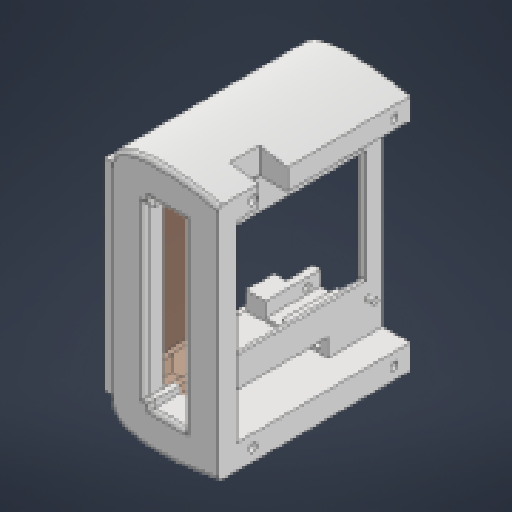
# Autodesk Inventor part: BP_BackHSCover
Saved by Autodesk Inventor 2026.1 (Build 301233020, 233B)
## iProperties
Created: 2025-09-12
Part Number: BP_BackHSCover
Material: Generic
Document SubType Name: Modeling
Designer: atrus
Density: 1 g/cm^3
Appearance: Default
Author: atrus
Autodesk Inventor part; units mm, degrees
ref_plane "YZ Plane" through (0, 0, 0) normal (1, 0, 0) x (0, 1, 0)
ref_plane "XZ Plane" through (0, 0, 0) normal (0, 1, 0) x (-1, 0, 0)
ref_plane "XY Plane" through (0, 0, 0) normal (0, 0, 1) x (1, 0, 0)
ref_plane "Work Plane1" through (0, 0, 0) normal (0, 0, 1) x (1, 0, 0)
sketch "Sketch1" plane through (0, 0, 0) normal (0, 0, 1) x (1, 0, 0)
  line L0 (-13.535, 44.65) -> (-5.515, 44.65)
  line L1 (-13.535, 37.45) -> (-13.535, 44.65)
  line L2 (-5.515, 44.65) -> (-5.515, 41.182512)
  line L3 (-5.515, 41.182512) -> (-2.515, 41.182512)
  line L4 (-2.515, 41.182512) -> (-2.515, 44.65)
  line L5 (-2.515, 44.65) -> (13.535, 44.65)
  line L6 (17.335, 46.4) -> (30.735, 46.4)
  line L7 (-13.535, -44.65) -> (-13.535, -37.45)
  line L8 (-5.515, -44.65) -> (-13.535, -44.65)
  line L9 (-2.515, -44.65) -> (-2.515, -41.182512)
  line L10 (-2.515, -41.182512) -> (-5.515, -41.182512)
  line L11 (-5.515, -41.182512) -> (-5.515, -44.65)
  line L12 (13.535, -44.65) -> (-2.515, -44.65)
  line L13 (30.735, -46.4) -> (17.335, -46.4)
  line L14 (17.135, 44.65) -> (17.135, 46.4)
  line L15 (17.135, 46.4) -> (17.335, 46.4)
  line L16 (17.335, 6.800735) -> (17.335, 46.4) construction
  line L17 (17.135, -44.65) -> (17.135, -46.4)
  line L18 (17.135, -46.4) -> (17.335, -46.4)
  line L19 (17.135, -44.65) -> (13.535, -44.65)
  line L20 (13.535, -44.65) -> (13.535, -22.65)
  line L21 (13.535, -22.65) -> (17.135, -22.65)
  line L22 (17.135, -22.65) -> (17.135, -44.65)
  line L23 (13.535, -22.65) -> (17.135, -22.65)
  line L24 (17.135, 44.65) -> (17.135, 32.65)
  line L25 (17.135, 32.65) -> (13.535, 32.65)
  line L26 (13.535, 32.65) -> (13.535, 44.65)
  spline S0 degree 3 poles (-23.335, 49.666) (-23.335, 50.975038) (-23.115819, 52.251766) (-22.162072, 54.544569) (-21.511946, 55.503776) (-19.686621, 57.40022) (-18.462391, 58.23491) (-14.911188, 60.065087) (-12.299571, 60.793194) (-3.902353, 62.358148) (2.96136, 62.289587) (16.161219, 61.311935) (23.649527, 60.13196) (30.735, 58.666) knots 0 0 0 0 0.39271137 0.39271137 0.74506577 0.74506577 1.1824292 1.1824292 1.94381451 1.94381451 3.74663198 3.74663198 5.90158117 5.90158117 5.90158117 5.90158117
  line L27 (30.735, 46.4) -> (30.735, 58.666)
  spline S1 degree 3 poles (30.735, -58.666) (16.274892, -61.657747) (2.749294, -62.920017) (-10.548387, -61.239744) (-14.259292, -60.426866) (-18.693704, -58.102852) (-20.021433, -57.155699) (-21.800919, -55.095353) (-22.369255, -54.150468) (-23.158123, -51.996135) (-23.335, -50.841944) (-23.335, -49.666) knots 0 0 0 0 4.42990689 4.42990689 5.93568564 5.93568564 6.64545407 6.64545407 7.1403284 7.1403284 7.66063661 7.66063661 7.66063661 7.66063661
  line L28 (30.735, -46.4) -> (30.735, -58.666)
  line L29 (-23.335, -37.45) -> (-13.535, -37.45)
  line L30 (-23.335, 37.45) -> (-13.535, 37.45)
  line L31 (-23.335, 49.666) -> (-23.335, 37.45)
  line L32 (-23.335, -37.45) -> (-23.335, -49.666)
  point P0 (0, 0)
  dimension "d0" = 0.2
  dimension "d13" = 22
  dimension "d15" = 3.6
  dimension "d16" = 12
  constraints: 24 end point, 4 parallel, 4 perpendicular, 2 collinear, 1 horizontal
  measures "d0" distance between parallel lines of L16 L14
  measures "d13" distance of L19.end L20.end
  measures "d15" distance between parallel lines of L22 L20
  measures "d16" distance from line of L5.end L25
extrude "Main" add sketch "Sketch1" against normal blind 80
sketch "Sketch2" plane through (0, 0, 0) normal (0, 0, 1) x (1, 0, 0)
  line L0 (17.335, 47.5) -> (18.75516, 47.5) construction
  line L1 (18.75516, 44.5) -> (18.75516, 47.5) construction
  line L2 (17.335, 47.5) -> (17.335, 44.5) construction
  line L3 (30.735, 44.216635) -> (30.735, 47.7)
  line L4 (30.735, 47.7) -> (17.135, 47.7)
  line L5 (17.135, 47.7) -> (17.135, 44.216635)
  line L6 (17.135, 44.216635) -> (30.735, 44.216635)
  line L7 (17.135, 32.65) -> (17.135, 46.4)
  point P0 (0, 0)
  point P1 (17.135, 44.65)
  point P2 (30.735, 46.4)
  dimension "d3" = 0.2
  constraints: 8 end point, 3 perpendicular, 1 collinear, 1 point on line, 1 vertical
  measures "d3" distance between parallel lines of L4 L0
extrude "PCBCut" cut sketch "Sketch2" against normal blind 80
sketch "Sketch3" plane through (17.135, 47.7, 0) normal (0, -1, 0) x (1, 0, 0)
  line L0 (4.55476, -15.371998) -> (4.55476, -8.992003) construction
  arc A0 (4.55476, -8.992003) -> (3.574762, -8.012) centre (3.57476, -8.992) ccw construction
  arc A1 (3.574761, -16.352) -> (4.55476, -15.371998) centre (3.57476, -15.372) ccw construction
  line L1 (1.62016, -77) -> (1.62016, 2) construction
  line L2 (2.62016, -5.012) -> (13.6, -5.012)
  line L3 (13.6, -5.012) -> (13.6, -19.352)
  line L4 (13.6, -19.352) -> (2.62016, -19.352)
  line L5 (1.62016, -18.352) -> (1.62016, -6.012)
  line L6 (13.6, 0) -> (13.6, -80) construction
  line L7 (13.6, 0) -> (13.6, -80)
  line L8 (1.62016, -6.012) -> (1.62016, -5.012)
  line L9 (2.62016, -5.012) -> (1.62016, -5.012)
  line L10 (1.62016, -18.352) -> (1.62016, -19.352)
  line L11 (2.62016, -19.352) -> (1.62016, -19.352)
  point P0 (-17.135, 0)
  point P1 (13.6, -12.182)
  dimension "d6" = 3
  dimension "d7" = 3
  constraints: 18 end point, 5 point on line, 2 horizontal, 2 parallel, 2 perpendicular, 1 collinear, 1 midpoint
  measures "d6" distance from line of L2 A0.end
  measures "d7" distance from line of L4 A1.start
extrude "USBCCut" cut sketch "Sketch3" against normal blind 80
sketch "Sketch4" plane through (0, 0, 0) normal (0, 0, 1) x (1, 0, 0)
  line L0 (17.135, 47.7) -> (30.735, 47.7)
  line L1 (-23.335, 49.666) -> (-23.335, 37.45)
  line L2 (-23.335, 37.45) -> (-13.535, 37.45)
  line L3 (-13.535, 37.45) -> (-13.535, 44.65)
  line L4 (-13.535, 44.65) -> (-5.515, 44.65)
  line L5 (-5.515, 44.65) -> (-5.515, 41.182512)
  line L6 (-5.515, 41.182512) -> (-2.515, 41.182512)
  line L7 (-2.515, 41.182512) -> (-2.515, 44.65)
  line L8 (-2.515, 44.65) -> (13.535, 44.65)
  line L9 (17.135, 32.65) -> (17.135, 47.7)
  line L10 (17.135, -22.65) -> (13.535, -22.65)
  line L11 (13.535, -22.65) -> (13.535, -44.65)
  line L12 (13.535, 44.65) -> (13.535, 32.65)
  line L13 (13.535, 32.65) -> (17.135, 32.65)
  line L14 (30.735, 47.7) -> (30.735, 58.666)
  spline S0 degree 3 poles (30.735, 58.666) (23.649527, 60.13196) (16.161219, 61.311935) (2.96136, 62.289587) (-3.902353, 62.358148) (-12.299571, 60.793194) (-14.911188, 60.065087) (-18.462391, 58.23491) (-19.686621, 57.40022) (-21.511946, 55.503776) (-22.162072, 54.544569) (-23.115819, 52.251766) (-23.335, 50.975038) (-23.335, 49.666) knots 0 0 0 0 0.36514777 0.36514777 0.67062818 0.67062818 0.79964197 0.79964197 0.8737515 0.8737515 0.93345658 0.93345658 1 1 1 1
  line L15 (13.535, -44.65) -> (-2.515, -44.65)
  line L16 (-2.515, -44.65) -> (-2.515, -41.182512)
  line L17 (-2.515, -41.182512) -> (-5.515, -41.182512)
  line L18 (-5.515, -41.182512) -> (-5.515, -44.65)
  line L19 (-5.515, -44.65) -> (-13.535, -44.65)
  line L20 (-13.535, -44.65) -> (-13.535, -37.45)
  line L21 (-13.535, -37.45) -> (-23.335, -37.45)
  line L22 (-23.335, -37.45) -> (-23.335, -49.666)
  spline S1 degree 3 poles (-23.335, -49.666) (-23.335, -50.841944) (-23.158123, -51.996135) (-22.369255, -54.150468) (-21.800919, -55.095353) (-20.021433, -57.155699) (-18.693704, -58.102852) (-14.259292, -60.426866) (-10.548387, -61.239744) (2.749294, -62.920017) (16.274892, -61.657747) (30.735, -58.666) knots 0 0 0 0 0.06791971 0.06791971 0.13251934 0.13251934 0.22517071 0.22517071 0.42173123 0.42173123 1 1 1 1
  line L23 (30.735, -58.666) -> (30.735, -46.4)
  line L24 (30.735, -46.4) -> (17.135, -46.4)
  line L25 (17.135, -46.4) -> (17.135, -22.65)
  point P0 (0, 0)
  constraints: 2 other
extrude "EndExt" add sketch "Sketch4" along normal blind 5.5
ref_plane "Work Plane2" through (0, 0, 0.2) normal (0, 0, 1) x (1, 0, 0)
sketch "Sketch7" plane through (0, 0, 5.5) normal (0, 0, 1) x (1, 0, 0)
  line L0 (-13.535, 37.45) -> (-13.535, 44.65)
  line L1 (-23.335, 37.45) -> (-13.535, 37.45)
  line L2 (-23.335, 46.4) -> (-23.335, 37.45)
  line L3 (-23.335, 46.4) -> (-1.335, 46.4)
  line L4 (-1.335, 46.4) -> (-1.335, 44.65)
  line L5 (-2.515, 44.65) -> (-1.335, 44.65)
  line L6 (-2.515, 41.182512) -> (-2.515, 44.65)
  line L7 (-5.515, 41.182512) -> (-2.515, 41.182512)
  line L8 (-5.515, 44.65) -> (-5.515, 41.182512)
  line L9 (-13.535, 44.65) -> (-5.515, 44.65)
  line L10 (30.735, 47.7) -> (30.735, 58.666)
  spline S0 degree 3 poles (30.735, 58.666) (23.649527, 60.13196) (16.161219, 61.311935) (2.96136, 62.289587) (-3.902353, 62.358148) (-12.299571, 60.793194) (-14.911188, 60.065087) (-18.462391, 58.23491) (-19.686621, 57.40022) (-21.511946, 55.503776) (-22.162072, 54.544569) (-23.115819, 52.251766) (-23.335, 50.975038) (-23.335, 49.666) knots 0 0 0 0 0.36514777 0.36514777 0.67062818 0.67062818 0.79964197 0.79964197 0.8737515 0.8737515 0.93345658 0.93345658 1 1 1 1
  line L11 (-23.335, 49.666) -> (-23.335, 37.45)
  line L12 (-23.335, 37.45) -> (-13.535, 37.45)
  line L13 (-13.535, 37.45) -> (-13.535, 44.65)
  line L14 (-13.535, 44.65) -> (-5.515, 44.65)
  line L15 (-5.515, 44.65) -> (-5.515, 41.182512)
  line L16 (-5.515, 41.182512) -> (-2.515, 41.182512)
  line L17 (-2.515, 41.182512) -> (-2.515, 44.65)
  line L18 (-2.515, 44.65) -> (13.535, 44.65)
  line L19 (13.535, 44.65) -> (13.535, 32.65)
  line L20 (13.535, 32.65) -> (17.135, 32.65)
  line L21 (17.135, 32.65) -> (17.135, 47.7)
  line L22 (17.135, 47.7) -> (30.735, 47.7)
  line L23 (13.535, -22.65) -> (13.535, -44.65)
  line L24 (13.535, -44.65) -> (-2.515, -44.65)
  line L25 (-2.515, -44.65) -> (-2.515, -41.182512)
  line L26 (-2.515, -41.182512) -> (-5.515, -41.182512)
  line L27 (-5.515, -41.182512) -> (-5.515, -44.65)
  line L28 (-5.515, -44.65) -> (-13.535, -44.65)
  line L29 (-13.535, -44.65) -> (-13.535, -37.45)
  line L30 (-13.535, -37.45) -> (-23.335, -37.45)
  line L31 (-23.335, -37.45) -> (-23.335, -49.666)
  spline S1 degree 3 poles (-23.335, -49.666) (-23.335, -50.841944) (-23.158123, -51.996135) (-22.369255, -54.150468) (-21.800919, -55.095353) (-20.021433, -57.155699) (-18.693704, -58.102852) (-14.259292, -60.426866) (-10.548387, -61.239744) (2.749294, -62.920017) (16.274892, -61.657747) (30.735, -58.666) knots 0 0 0 0 0.06791971 0.06791971 0.13251934 0.13251934 0.22517071 0.22517071 0.42173123 0.42173123 1 1 1 1
  line L32 (30.735, -58.666) -> (30.735, -46.4)
  line L33 (30.735, -46.4) -> (17.135, -46.4)
  line L34 (17.135, -46.4) -> (17.135, -22.65)
  line L35 (17.135, -22.65) -> (13.535, -22.65)
  line L36 (-5.515, 41.182512) -> (-5.515, -41.182512)
  line L37 (-23.335, 37.45) -> (-23.335, -37.45)
  line L38 (13.535, 32.65) -> (13.535, -22.65)
  line L39 (30.735, 47.7) -> (30.735, -46.4)
  constraints: 8 end point, 2 parallel, 2 vertical, 2 other
extrude "Endcap" add sketch "Sketch7" along normal blind 9 contours L1 L2 L3 L4 L5 L6 L7 L8 L9 L0 | L0 L9 L8 L36 L27 L28 L29 L30 L37 L1 | L11 S0 L10 L22 L21 L20 L19 L18 L4 L3 | L30 L29 L28 L27 L26 L25 L24 L23 L35 L34 L33 L32 S1 L31 | L39 L33 L34 L35 L38 L20 L21 L22
fillet "Fillet1" radius 2 10 edges at (-23.335, 0, 14.5) (-2.9539, -62.0389, 14.5) (0.6695, 62.1456, 14.5) (13.535, 0, 14.5) (5.51, 44.65, 14.5) (-2.515, 42.9163, 14.5) (-4.015, 41.1825, 14.5) (-5.515, 0, 14.5) (-4.015, -41.1825, 14.5) (5.51, -44.65, 14.5)
sketch "Sketch8" plane through (17.135, -46.4, -80) normal (1, 0, 0) x (0, 0, -1)
  line L0 (0, 0) -> (-80.2, 0) projected
  line L1 (0, 8.95) -> (-80.2, 8.95) projected
  line L2 (-73.2, 0) -> (-27, 0)
  line L3 (-27, 0) -> (-27, 8.95)
  line L4 (-27, 8.95) -> (-73.2, 8.95)
  line L5 (-73.2, 8.95) -> (-73.2, 0)
  line L6 (-80.2, 0) -> (-80.2, 94.1) projected
  line L7 (0, 23.75) -> (0, 0) projected
  point P0 (-80, 46.4)
  point P1 (-27, 4.475)
  point P2 (-73.2, 8.95)
  dimension "d21" = 7
  dimension "d22" = 27
  constraints: 8 end point, 2 parallel, 2 point on line, 1 horizontal, 1 midpoint, 1 perpendicular
  measures "d21" distance between parallel lines of L6 L5
  measures "d22" distance from line of L7 point (-27, 4.475)
extrude "CutCord1" cut sketch "Sketch8" against normal blind 45 contours L0 L5 L1 L3
sketch "Sketch9" plane through (-23.335, -49.666, -80) normal (-1, 0, 0) x (0, 0, 1)
  line L0 (73.2, 87.116) -> (27, 87.116)
  line L1 (27, 87.116) -> (27, 96.066)
  line L2 (27, 96.066) -> (73.2, 96.066)
  line L3 (73.2, 96.066) -> (73.2, 87.116)
  line L4 (0, 87.116) -> (80.2, 87.116) projected
  line L5 (27, 3.266) -> (27, 12.216) projected
  line L6 (73.2, 12.216) -> (73.2, 3.266) projected
  point P0 (80, 49.666)
  point P1 (73.2, 91.591)
  dimension "d68" = 7
  constraints: 8 end point, 3 collinear, 2 parallel, 1 horizontal, 1 midpoint, 1 perpendicular
  measures "d68" horizontal distance of L4.end point (73.2, 91.591)
extrude "CutCord2" cut sketch "Sketch9" against normal blind 22
sketch "Sketch10" plane through (0, 0, 14.5) normal (0, 0, 1) x (1, 0, 0)
  line L0 (-5.515, 41.182512) -> (-2.515, 41.182512)
  line L1 (-6.815, -44.65) -> (-6.815, 44.65)
  line L2 (-2.515, 41.182512) -> (-6.815, 41.182512)
  line L3 (-6.815, 41.182512) -> (-6.815, 44.65)
  line L4 (-6.815, 44.65) -> (-2.515, 44.65)
  line L5 (-2.515, 44.65) -> (-2.515, 41.182512)
  line L6 (-2.515, -41.182512) -> (-5.515, -41.182512)
  line L7 (-5.515, -44.65) -> (-13.535, -44.65)
  line L8 (-2.515, -41.182512) -> (-6.815, -41.182512)
  line L9 (-6.815, -41.182512) -> (-6.815, -44.65)
  line L10 (-6.815, -44.65) -> (-2.515, -44.65)
  line L11 (-2.515, -44.65) -> (-2.515, -41.182512)
  point P0 (0, 0)
  constraints: 16 end point, 4 parallel, 2 horizontal, 2 perpendicular, 2 point on line
extrude "Extrusion8" add sketch "Sketch10" against normal up to surface (9 mm away)
fillet "Fillet2" radius 2 6 edges at (-2.515, 42.9163, 14.5) (-4.665, 41.1825, 14.5) (-4.665, -41.1825, 14.5) (-2.515, -43.9163, 14.5) (13.535, 32.65, -37.25) (13.535, -22.65, -37.25)
sketch "Sketch12" plane through (30.735, -48.4, 0.2) normal (1, 0, 0) x (0, 0, -1)
  circle A0 centre (4.24, 93.4) radius 0.508
  circle A1 centre (1.7, 93.4) radius 0.508
  circle A2 centre (73.45, 17.65) radius 1.799996
  circle A3 centre (1.95, 17.65) radius 1.799996
  circle A4 centre (73.45, 89.15) radius 1.799996
  circle A5 centre (1.95, 89.15) radius 1.799996
  circle A6 centre (15.272, 90.786) radius 0.325006
  circle A7 centre (9.492, 90.786) radius 0.325006
  arc A8 (7.762, 94.066) -> (8.362, 94.066) centre (8.062, 94.066) ccw
  line L0 (7.762, 94.066) -> (7.762, 94.866)
  arc A9 (8.362, 94.866) -> (7.762, 94.866) centre (8.062, 94.866) ccw
  line L1 (8.362, 94.866) -> (8.362, 94.066)
  arc A10 (16.402, 94.066) -> (17.002, 94.066) centre (16.702, 94.066) ccw
  line L2 (16.402, 94.066) -> (16.402, 94.866)
  arc A11 (17.002, 94.866) -> (16.402, 94.866) centre (16.702, 94.866) ccw
  line L3 (17.002, 94.866) -> (17.002, 94.066)
  arc A12 (7.762, 89.736) -> (8.362, 89.736) centre (8.062, 89.736) ccw
  line L4 (7.762, 89.736) -> (7.762, 90.836)
  arc A13 (8.362, 90.836) -> (7.762, 90.836) centre (8.062, 90.836) ccw
  line L5 (8.362, 90.836) -> (8.362, 89.736)
  arc A14 (16.402, 89.736) -> (17.002, 89.736) centre (16.702, 89.736) ccw
  line L6 (16.402, 89.736) -> (16.402, 90.836)
  arc A15 (17.002, 90.836) -> (16.402, 90.836) centre (16.702, 90.836) ccw
  line L7 (17.002, 90.836) -> (17.002, 89.736)
  circle A16 centre (44.2, 75.9) radius 0.625005
  circle A17 centre (46.74, 73.74) radius 0.509994
  circle A18 centre (44.2, 73.74) radius 0.509994
  circle A19 centre (41.66, 73.74) radius 0.509994
  circle A20 centre (39.12, 73.74) radius 0.509994
  circle A21 centre (67.002, 89.87) radius 0.509994
  circle A22 centre (67.002, 86.87) radius 0.509994
  circle A23 centre (64.002, 89.87) radius 0.509994
  circle A24 centre (64.002, 86.87) radius 0.509994
  circle A25 centre (63.062, 83.87) radius 0.509994
  circle A26 centre (63.062, 92.87) radius 0.509994
  line L8 (-1.8, 10.9) -> (77.2, 10.9)
  arc A27 (77.2, 10.9) -> (80.2, 13.9) centre (77.199999, 13.900001) ccw
  line L9 (80.2, 13.9) -> (80.2, 92.9)
  arc A28 (80.2, 92.9) -> (77.2, 95.9) centre (77.199999, 92.899999) ccw
  line L10 (77.2, 95.9) -> (-1.8, 95.9)
  arc A29 (-1.8, 95.9) -> (-4.8, 92.9) centre (-1.799999, 92.899999) ccw
  line L11 (-4.8, 92.9) -> (-4.8, 13.9)
  arc A30 (-4.8, 13.9) -> (-1.8, 10.9) centre (-1.799999, 13.900001) ccw
  line L12 (-1.799999, 96.7) -> (77.199999, 96.7)
  arc A31 (81, 92.899999) -> (77.199999, 96.7) centre (77.199999, 92.899999) ccw
  line L13 (81, 92.899999) -> (81, 13.900001)
  arc A32 (77.199999, 10.1) -> (81, 13.900001) centre (77.199999, 13.900001) ccw
  line L14 (77.199999, 10.1) -> (-1.799999, 10.1)
  arc A33 (-5.6, 13.900001) -> (-1.799999, 10.1) centre (-1.799999, 13.900001) ccw
  line L15 (-5.6, 13.900001) -> (-5.6, 92.899999)
  arc A34 (-1.799999, 96.7) -> (-5.6, 92.899999) centre (-1.799999, 92.899999) ccw
  dimension "d86" = 0.8
  constraints: 8 end point, 8 point on circle, 4 centre point, 7 other
  measures "d86" distance between parallel lines of L10 L12
extrude "EdgePCBCut" cut sketch "Sketch12" against normal up to surface (13.6 mm away) contours A0 | A1 | A2 | A3 | A4 | A5 | A6 | A7 | L0 A9 L1 A8 | L2 A11 L3 A10 | L4 A13 L5 A12 | L6 A15 L7 A14 | A16 | A17 | A18 | A19 | A20 | A21 | A22 | A23 | A24 | A25 | A26 | A30 L11 A29 L10 A28 L9 A27 L8 | L12 A31 L13 A32 L14 A33 L15 A34
sketch "Sketch13" plane through (17.135, -46.4, -80) normal (1, 0, 0) x (0, 0, -1)
  line L0 (-9, 93.9) -> (-20, 93.9)
  line L1 (-20, 93.9) -> (-20, 80.9)
  line L2 (-20, 80.9) -> (-9, 80.9)
  line L3 (-9, 80.9) -> (-9, 93.9)
  line L4 (0, 94.1) -> (0, 79.05) projected
  line L5 (-3, 93.9) -> (-82, 93.9) projected
  line L6 (-3, 93.9) -> (-82, 93.9) projected
  point P0 (-80, 46.4)
  point P1 (-14.5, 93.9)
  dimension "d39" = 13
  dimension "d40" = 9
  dimension "d41" = 11
  constraints: 8 end point, 2 parallel, 1 horizontal, 1 midpoint, 1 perpendicular, 1 point on line
  measures "d39" distance of L2.end L0.start
  measures "d40" distance between parallel lines of L4 L3
  measures "d41" distance of L1.end L2.end
extrude "PowerPinsCutout" cut sketch "Sketch13" against normal blind 10
sketch "Sketch11" plane through (17.135, -46.4, -80) normal (1, 0, 0) x (0, 0, -1)
  circle A0 centre (-6.75, 87.15) radius 1.799996 construction
  circle A1 centre (-78.25, 87.15) radius 1.799996 construction
  circle A2 centre (-78.25, 15.65) radius 1.799996 construction
  circle A3 centre (-6.75, 15.65) radius 1.799996 construction
  circle A4 centre (-6.75, 87.15) radius 1.699996
  circle A5 centre (-6.75, 15.65) radius 1.699996
  circle A6 centre (-78.25, 87.15) radius 1.699996
  circle A7 centre (-78.25, 15.65) radius 1.699996
  point P0 (-80, 46.4)
  dimension "d33" = 0.1
  constraints: 4 centre point, 4 coincident, 3 equal radius
  measures "d33" radial gap between concentric circles of A4 A0
extrude "PCBBoss" add sketch "Sketch11" along normal blind 3
sketch "Sketch14" plane through (0, 0, -80) normal (0, 0, -1) x (-1, 0, 0)
  arc A0 (-15.535, 32.65) -> (-13.535, 34.65) centre (-15.535, 34.65) ccw projected
  line L0 (-17.135, -22.65) -> (-17.135, -46.4) projected
  line L1 (-13.535, 34.65) -> (-17.135, 34.65)
  line L2 (-17.135, 34.65) -> (-17.135, -24.65)
  line L3 (-17.135, -24.65) -> (-13.535, -24.65)
  line L4 (-13.535, -24.65) -> (-13.535, 34.65)
  point P0 (0, 0)
  constraints: 8 end point, 2 parallel, 1 horizontal, 1 perpendicular, 1 point on circle, 1 point on line
extrude "Extrusion12" add sketch "Sketch14" against normal blind 8
fillet "Fillet4" radius 2 3 edges at (13.535, 39.6499, -80) (13.535, 5, -80) (13.535, -34.6499, -80)
sketch "Sketch15" plane through (-23.335, -49.666, -80) normal (-1, 0, 0) x (0, 0, 1)
  line L0 (0, 12.216) -> (80.2, 12.216) projected
  line L1 (0, 0) -> (85.5, 0) projected
  line L2 (0, 12.216) -> (13, 12.216)
  line L3 (13, 12.216) -> (13, 0)
  line L4 (13, 0) -> (0, 0)
  line L5 (0, 0) -> (0, 12.216)
  line L6 (85.5, 87.116) -> (0, 87.116) projected
  line L7 (0, 99.332) -> (92.5, 99.332) projected
  line L8 (0, 87.116) -> (13, 87.116)
  line L9 (13, 87.116) -> (13, 99.332)
  line L10 (13, 99.332) -> (0, 99.332)
  line L11 (0, 99.332) -> (0, 87.116)
  point P0 (80, 49.666)
  point P1 (27, 12.216)
  point P2 (27, 87.116)
  point P3 (85.5, 99.332)
  point P4 (0, 6.108)
  point P5 (13, 87.116)
  point P6 (13, 12.216)
  point P7 (94.5, 99.332)
  dimension "d48" = 13
  constraints: 16 end point, 4 parallel, 2 horizontal, 2 perpendicular, 2 point on line, 1 collinear, 1 midpoint
  measures "d48" distance from line of point (0, 6.108) L3
extrude "Extrusion13" cut sketch "Sketch15" against normal blind 6
sketch "Sketch16" plane through (-17.335, -49.666, -80) normal (-1, 0, 0) x (0, 0, 1)
  line L0 (13, 0) -> (0, 0) construction
  line L1 (6.5, 0) -> (7.78824, 99.332) construction
  line L2 (0, 99.332) -> (92.5, 99.332) construction
  line L3 (0, 12.216) -> (13, 12.216)
  line L4 (13, 87.116) -> (0, 87.116)
  point P0 (80, 49.666)
  point P1 (13, 99.332)
  point P2 (7.688171, 91.616)
  point P3 (6.600069, 7.716)
  point P4 (85.5, 99.332)
  point P5 (94.5, 99.332)
  dimension "d51" = 4.5
  dimension "d52" = 4.5
  constraints: 3 point on line, 2 end point, 1 midpoint
  measures "d51" distance from line of L3 point (6.6, 7.716)
  measures "d52" distance from line of L4 point (7.688, 91.616)
hole "Hole1" at (-17.335, 41.95, -72.311829) at (-17.335, -41.95, -73.399931) direction (1, 0, 0) diameter 3.6 depth 8 tip angle 118 clearance for "Flat Head Machine Screw" size "M3" standard "Ansi Metric M Profile"
sketch "Sketch17" plane through (0, 0, -80) normal (0, 0, -1) x (-1, 0, 0)
  line L0 (17.335, 45.65) -> (17.335, 49.666) projected
  line L1 (13.335, 45.65) -> (17.335, 45.65) projected
  line L2 (13.335, 48.65) -> (13.335, 45.65) projected
  line L3 (-29.735, 48.65) -> (13.335, 48.65) projected
  line L4 (-29.735, 52.65) -> (-29.735, 48.65) projected
  line L5 (17.335, 52.65) -> (-29.735, 52.65) projected
  line L6 (17.335, 49.666) -> (17.335, 52.65) projected
  line L7 (17.335, -45.65) -> (13.335, -45.65) projected
  line L8 (17.335, -49.666) -> (17.335, -45.65) projected
  line L9 (17.335, -52.65) -> (17.335, -49.666) projected
  line L10 (-29.735, -52.65) -> (17.335, -52.65) projected
  line L11 (-29.735, -48.65) -> (-29.735, -52.65) projected
  line L12 (13.335, -48.65) -> (-29.735, -48.65) projected
  line L13 (13.335, -45.65) -> (13.335, -48.65) projected
  point P0 (0, 0)
extrude "Extrusion14" cut sketch "Sketch17" against normal blind 2
sketch "Sketch18" plane through (30.735, -58.666, -80) normal (1, 0, 0) x (0, 0, -1)
  line L0 (0, 10.266) -> (-85.5, 10.266) construction
  line L1 (0, 0) -> (-85.5, 0) construction
  line L2 (0, 12.266) -> (0, 0) construction
  line L3 (0, 6.133) -> (-85.5, 6.133) construction
  line L4 (-60.648, 117.332) -> (0, 117.332) construction
  line L5 (-60.648, 106.366) -> (0, 106.366) construction
  line L6 (0, 117.332) -> (0, 106.366) construction
  line L7 (0, 111.849) -> (-85.5, 111.849) construction
  circle A0 centre (-8, 6.133) radius 2
  circle A1 centre (-77.5, 6.133) radius 2
  circle A2 centre (-8, 111.849) radius 2
  circle A3 centre (-77.5, 111.849) radius 2
  line L8 (-85.5, 0) -> (-85.5, 9) projected
  point P0 (-80, 58.666)
  point P1 (-85.5, 12.266)
  dimension "d62" = 8
  dimension "d63" = 8
  dimension "d64" = 4
  constraints: 5 point on line, 4 centre point, 4 end point, 3 equal radius, 2 horizontal, 2 midpoint, 2 vertical alignment
  measures "d62" distance from line of L2 A0.centre
  measures "d63" distance of L3.end A1.centre
  measures "d64" diameter of A0
extrude "Extrusion15" cut sketch "Sketch18" against normal blind 7
sketch "Sketch20" plane through (-23.335, -37.45, 5.5) normal (-1, 0, 0) x (0, 0, 1)
  line L0 (-72.5, 87.116) -> (-72.5, 74.9) construction
  line L1 (-58.5, 74.9) -> (-72.5, 74.9) construction
  line L2 (-58.5, 74.9) -> (-58.5, 83.85) construction
  line L3 (-58.5, 83.85) -> (-12.3, 83.85) construction
  line L4 (-12.3, 83.85) -> (-12.3, 74.9) construction
  line L5 (0, 74.9) -> (-12.3, 74.9) construction
  line L6 (-72.5, 87.116) -> (7, 87.116) construction
  line L7 (-67.2, -12.216) -> (7, -12.216)
  line L8 (-67.2, -12.216) -> (7, -12.216) projected
  line L9 (9, 87.116) -> (7, 87.116) projected
  line L10 (7, 87.116) -> (-72.5, 87.116)
  line L11 (7, -12.216) -> (7, 87.116)
  line L12 (-72.5, 87.116) -> (-72.5, 85.316)
  line L13 (5.2, 85.316) -> (5.2, -10.416)
  line L14 (5.2, -10.416) -> (-67.2, -10.416)
  line L15 (-67.2, -12.216) -> (-67.2, -10.416)
  line L16 (-72.5, 85.316) -> (5.2, 85.316)
  line L17 (0, 74.9) -> (0, 0) projected
  line L18 (-12.3, 0) -> (0, 0) projected
  line L19 (-12.3, 0) -> (-12.3, -8.95) projected
  line L20 (-12.3, -8.95) -> (-58.5, -8.95) projected
  line L21 (-58.5, -8.95) -> (-58.5, 0) projected
  line L22 (-72.5, 0) -> (-58.5, 0) projected
  line L23 (-72.5, 0) -> (-72.5, -12.216) projected
  line L24 (-72.5, -12.216) -> (7, -12.216) projected
  line L25 (7, 87.116) -> (7, -12.216) projected
  point P0 (-5.5, 37.45)
  point P1 (5.3, -12.216)
  point P2 (9, -12.216)
  dimension "d74" = 1.8
  dimension "d76" = 1.8
  constraints: 16 end point, 3 perpendicular, 1 collinear, 1 point on line
  measures "d74" distance between parallel lines of L6 L16
  measures "d76" distance between parallel lines of L7 L14
extrude "Extrusion17" add sketch "Sketch20" along normal blind 4
sketch "Sketch21" plane through (-23.335, -37.45, 5.5) normal (-1, 0, 0) x (0, 0, 1)
  circle A0 centre (-3.5, -3.5) radius 1.9
  circle A1 centre (-3.5, 78.4) radius 1.9
  arc A2 (-5.5, -2.456367) -> (-5.5, -4.543633) centre (-6.15, -3.5) ccw
  arc A3 (-5.5, 79.443633) -> (-5.5, 77.356367) centre (-6.15, 78.4) ccw
  point P0 (-5.5, 37.45)
  dimension "d79" = 3.8
  dimension "d80" = 3.8
  constraints: 2 centre point
  measures "d79" diameter of A1
  measures "d80" diameter of A0
extrude "Extrusion18" cut sketch "Sketch21" against normal blind 10
sketch "Sketch22" plane through (18.75516, 47.7, -6.012) normal (1, 0, 0) x (0, 0, -1)
  line L0 (-1, 0.6) -> (13.34, 0.6)
  line L1 (13.34, 0.6) -> (13.34, 13.070874)
  spline S0 degree 6 poles (-1, 13.070874) (-0.833333, 13.070874) (-0.666667, 13.070874) (-0.5, 13.070874) (-0.333333, 13.070874) (-0.166667, 13.070874) (1.591281, 13.070874) (3.753455, 13.070874) (6.260891, 13.070874) (8.874675, 13.070874) (11.166431, 13.070874) (12.506667, 13.070874) (12.673333, 13.070874) (12.84, 13.070874) (13.006667, 13.070874) (13.173333, 13.070874) (13.34, 13.070874) knots 0 0 0 0 0 0 0 0.08400808 0.08400808 0.08400808 0.08400808 0.08400808 0.8860907 0.8860907 0.8860907 0.8860907 0.8860907 1 1 1 1 1 1 1
  line L2 (-1, 0.6) -> (-1, 13.070874)
  line L3 (13.34, 13.070874) -> (-1, 13.070874)
  line L4 (-1, 13.070874) -> (-1, 35.697177)
  line L5 (-1, 35.697177) -> (13.34, 35.697177)
  line L6 (13.34, 35.697177) -> (13.34, 13.070874)
  point P0 (-6.012, -47.7)
  constraints: 8 end point, 2 parallel, 1 horizontal, 1 perpendicular, 1 other
extrude "Extrusion19" cut sketch "Sketch22" against normal blind 2
body "Solid1"
